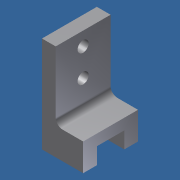
# Autodesk Inventor part: gripper jaw
Saved by Autodesk Inventor 2012 (Build 160160000, 160)
## iProperties
Created: 2012-07-09
Part Number: gripper jaw
Material: Default
Document SubType Name: Modeling
Designer: Ed
Density: 1 g/cm^3
Author: Ed
Autodesk Inventor part; units mm, degrees
ref_plane "YZ Plane" through (0, 0, 0) normal (1, 0, 0) x (0, 1, 0)
ref_plane "XZ Plane" through (0, 0, 0) normal (0, 1, 0) x (-1, 0, 0)
ref_plane "XY Plane" through (0, 0, 0) normal (0, 0, 1) x (1, 0, 0)
sketch "Sketch1" plane through (0, 0, 0) normal (0, 0, 1) x (1, 0, 0)
  line L0 (0, 0) -> (19.05, 0)
  line L1 (19.05, 0) -> (19.05, 44.45)
  line L2 (19.05, 44.45) -> (0, 44.45)
  line L3 (0, 44.45) -> (0, 0)
  line L4 (19.05, 44.45) -> (6.35, 44.45)
  line L5 (6.35, 44.45) -> (6.35, 15.875)
  line L6 (9.525, 12.7) -> (19.05, 12.7)
  line L7 (19.05, 12.7) -> (19.05, 44.45)
  arc A0 (6.35, 15.875) -> (9.525, 12.7) centre (9.525, 15.875) ccw
  point P0 (6.35, 12.7)
  dimension "d0" = 44.45
  dimension "d1" = 19.05
  dimension "d2" = 31.75
  dimension "d3" = 6.35
  dimension "d4" = 3.175
  constraints: 16 end point, 4 parallel, 2 horizontal, 2 perpendicular, 2 point on circle, 2 point on line, 2 tangent, 1 centre point
  measures "d0" distance of L2.end L0.start
  measures "d1" distance of L0.start L0.end
  measures "d2" distance of L4.end point (6.35, 12.7)
  measures "d3" distance between parallel lines of L5 L3
  measures "d4" radius of A0
extrude "Extrusion1" add sketch "Sketch1" along normal blind 25.4 contours L3 L2 L5 A0 L6 L1 L0
sketch "Sketch2" plane through (0, 0, 0) normal (-1, 0, 0) x (0, 0, 1)
  line L0 (0, 44.45) -> (25.4, 44.45) projected
  point P0 (12.7, 38.1)
  point P1 (12.7, 25.4)
  point P2 (12.7, 44.45)
  dimension "d7" = 12.7
  dimension "d8" = 6.35
  constraints: 2 vertical alignment, 1 midpoint
  measures "d7" distance of point (12.7, 25.4) point (12.7, 38.1)
  measures "d8" distance of point (12.7, 44.45) point (12.7, 38.1)
hole "Hole1" at (0, 38.1, 12.7) at (0, 25.4, 12.7) direction (1, 0, 0) diameter 5.1054 end through all clearance for "Flat Head Machine Screw (82)" size "#10" standard "Ansi Unified Screw Threads"
sketch "Sketch3" plane through (0, 0, 0) normal (-1, 0, 0) x (0, 0, 1)
  line L0 (0, 0) -> (25.4, 0) projected
  line L1 (6.35, 0) -> (19.05, 0)
  line L2 (19.05, 0) -> (19.05, 7.62)
  line L3 (19.05, 7.62) -> (6.35, 7.62)
  line L4 (6.35, 7.62) -> (6.35, 0)
  point P0 (12.7, 0)
  dimension "d16" = 12.7
  dimension "d17" = 7.62
  constraints: 8 end point, 2 midpoint, 2 parallel, 1 horizontal, 1 perpendicular, 1 point on line
  measures "d16" distance of L2.end L3.end
  measures "d17" distance of L1.end L2.end
extrude "Extrusion2" cut sketch "Sketch3" against normal through all
body "Solid1"
